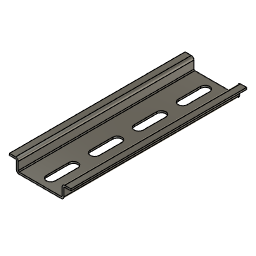
Parametric DIN Rail (Autodesk Fusion 360 design; units mm, degrees)
Autodesk Fusion 360 part; units mm, degrees
sketch "Skizze1" plane through (0, 0, 0) normal (0, 1, 0) x (1, 0, 0)
  line L0 (13.5, -1) -> (-13.5, -1)
  line L1 (-13.5, -1) -> (-13.5, 0)
  line L2 (-13.5, 0) -> (13.5, 0)
  line L3 (13.5, 0) -> (13.5, -1)
  line L4 (13.5, -1) -> (-13.5, 0) construction
  line L5 (-13.5, -1) -> (13.5, 0) construction
  line L6 (-13.5, 0) -> (-12.5, 0)
  line L7 (-12.5, 0) -> (-12.5, -7.5)
  line L8 (-12.5, -7.5) -> (-13.5, -7.5)
  line L9 (-13.5, -7.5) -> (-13.5, 0)
  line L10 (13.5, 0) -> (12.5, 0)
  line L11 (12.5, 0) -> (12.5, -7.5)
  line L12 (12.5, -7.5) -> (13.5, -7.5)
  line L13 (13.5, -7.5) -> (13.5, 0)
  line L14 (-12.5, -7.5) -> (-17.5, -7.5)
  line L15 (-17.5, -7.5) -> (-17.5, -6.5)
  line L16 (-17.5, -6.5) -> (-12.5, -6.5)
  line L17 (-12.5, -6.5) -> (-12.5, -7.5)
  line L18 (12.5, -7.5) -> (17.5, -7.5)
  line L19 (17.5, -7.5) -> (17.5, -6.5)
  line L20 (17.5, -6.5) -> (12.5, -6.5)
  line L21 (12.5, -6.5) -> (12.5, -7.5)
  point P0 (0, -0.5)
  dimension "d7" = 27
  dimension "d8" = 1
  dimension "d9" = 7.5
  dimension "d10" = 1
  dimension "d11" = 7.5
  dimension "d12" = 1
  dimension "d13" = 5
  dimension "d14" = 1
  dimension "d15" = 5
  dimension "d16" = 1
  constraint perpendicular L0 L1
  constraint parallel L0 L2
  constraint parallel L1 L3
  constraint horizontal L0
  constraint coincident L4 P0
  constraint coincident L5 P0
  constraint horizontal L6
  constraint vertical L7
  constraint horizontal L8
  constraint vertical L9
  constraint horizontal L10
  constraint vertical L11
  constraint horizontal L12
  constraint vertical L13
  constraint horizontal L14
  constraint vertical L15
  constraint horizontal L16
  constraint vertical L17
  constraint horizontal L18
  constraint vertical L19
  constraint horizontal L20
  constraint vertical L21
  measures "d7" distance of L1.end L2.end
  measures "d8" distance of L0.end L1.end
  measures "d9" distance of L1.end L8.end
  measures "d10" distance of L1.end L6.end
  measures "d11" distance of L2.end L12.end
  measures "d12" distance of L2.end L10.end
  measures "d13" distance of L7.end L14.end
  measures "d14" distance of L7.end L16.end
  measures "d15" distance of L11.end L18.end
  measures "d16" distance of L11.end L20.end
extrude "Extrusion1" add sketch "Skizze1" along normal blind 100
fillet "Abrundung1" radius 1.5 4 edges at (12.5, 50, 7.5) (-12.5, 50, 7.5) (13.5, 50, 0) (-13.5, 50, 0)
fillet "Abrundung2" radius 0.5 4 edges at (-13.5, 50, 6.5) (13.5, 50, 6.5) (12.5, 50, 1) (-12.5, 50, 1)
sketch "Skizze2" plane through (0, 0, 1) normal (0, 0, 1) x (-1, 0, 0)
  line L0 (12, -100) -> (12, 0)
  line L1 (12, 0) -> (-12, 0)
  line L2 (-12, 0) -> (-12, -100)
  line L3 (-12, -100) -> (12, -100)
  line L4 (0, 0) -> (0, -3.5) construction
  line L5 (-2.6, -6.1) -> (-2.6, -18.9)
  arc A0 (-2.6, -18.9) -> (2.6, -18.9) centre (0, -18.9) ccw
  line L6 (2.6, -18.9) -> (2.6, -6.1)
  arc A1 (2.6, -6.1) -> (-2.6, -6.1) centre (0, -6.1) ccw
  line L7 (0, -3.5) -> (0, -21.5) construction
  point P0 (0, -3.5)
  dimension "d26" = 3.5
  dimension "d34" = 18
  dimension "d35" = 5.2
  constraint coincident L4.start origin
  constraint perpendicular L3 L4
  constraint coincident P0 L4.end
  constraint tangent L5 A0
  constraint tangent A0 L6
  constraint parallel L5 L6
  constraint tangent L6 A1
  constraint tangent L5 A1
  constraint midpoint P0 A1
  constraint midpoint A0 L7.end
  constraint parallel L4 L7
  measures "d26" distance of L4.start P0
  measures "d34" distance of P0 L7.end
  measures "d35" diameter of A0
extrude "Extrusion2" cut sketch "Skizze2" against normal blind 1 contours L5 A0 L6 A1
pattern_linear "R-Anordnung1" count 4 spacing 25 along (0, 1, 0) of "Extrusion2"
equation "InnerWidth = 27 mm" comment "BI"
equation "OuterWidth = 37 mm" comment "Equals 35"
equation "Height = 7.5 mm" comment "h"
equation "Thickness = 1 mm" comment "D"
equation "Length = 100 mm" comment "L"
equation "SlotDistance = 25 mm" comment "ALL"
equation "d7 = InnerWidth"
equation "d8 = Thickness"
equation "d9 = Height"
equation "d10 = Thickness"
equation "d11 = Height"
equation "d12 = Thickness"
equation "d13 = ( OuterWidth - InnerWidth ) / 2"
equation "d14 = Thickness"
equation "d15 = ( OuterWidth - InnerWidth ) / 2"
equation "d16 = Thickness"
equation "d17 = Length"
equation "OuterFillet = 1.5 mm" comment "R"
equation "d20 = OuterFillet"
equation "InnerFillet = OuterFillet - Thickness" comment "RK"
equation "d22 = InnerFillet"
equation "SlotWidth = 5.2 mm" comment "LLB"
equation "SlotLength = 18 mm" comment "LLH"
equation "SlotDistance2 = 25 mm" comment "LLA"
equation "d26 = ( ( Length - ( ( Length / SlotDistance2 ) * SlotLength ) ) / ( Length / SlotDistance2 ) ) / 2"
equation "d28 = -Thickness"
equation "d30 = Length / SlotDistance2"
equation "d32 = SlotDistance2"
equation "d34 = SlotLength"
equation "d35 = SlotWidth"
